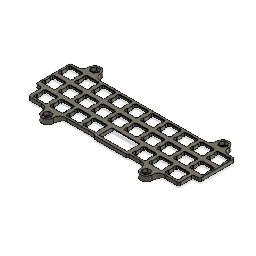
Alpha28PlateCase5mm v2 (Autodesk Fusion 360 design; units mm, degrees)
Autodesk Fusion 360 part; units mm, degrees
(part 1 of 6)
sketch "507b0d95479bd4c2c9a2277e45e886c67266d565_switch" plane through (0, 0, 0) normal (0, 1, 0) x (1, 0, 0)
  line L0 (189.063, 0.3128) -> (188.908, 0.2811)
  line L1 (190.215, 56.5838) -> (190.302, 56.4526)
  line L2 (190.444, 56.1728) -> (190.499, 56.0268)
  line L3 (189.063, 57.3525) -> (189.214, 57.3098)
  line L4 (1.3298, 0.4093) -> (1.1879, 0.474)
  line L5 (1.1879, 0.474) -> (1.0501, 0.5512)
  line L6 (1.6288, 0.3128) -> (1.4759, 0.3542)
  line L7 (190.302, 56.4526) -> (190.379, 56.315)
  line L8 (189.504, 57.1899) -> (189.64, 57.113)
  line L9 (190.444, 1.491) -> (190.379, 1.3491)
  line L10 (1.0501, 0.5512) -> (0.9192, 0.638)
  line L11 (190.572, 1.9444) -> (190.54, 1.7901)
  line L12 (190.117, 0.9577) -> (190.011, 0.842)
  line L13 (0.7965, 0.7359) -> (0.6808, 0.842)
  line L14 (0.5746, 0.9577) -> (0.4768, 1.0818)
  line L15 (0.248, 1.491) -> (0.1929, 1.6385)
  line L16 (1.4759, 0.3542) -> (1.3298, 0.4093)
  line L17 (189.771, 57.0258) -> (189.895, 56.9281)
  line L18 (0.4768, 1.0818) -> (0.39, 1.2127)
  line L19 (0.9192, 0.638) -> (0.7965, 0.7359)
  line L20 (190.499, 1.6385) -> (190.444, 1.491)
  line L21 (189.771, 0.638) -> (189.64, 0.5512)
  line L22 (190.572, 55.7209) -> (190.59, 55.5639)
  line L23 (190.379, 56.315) -> (190.444, 56.1728)
  line L24 (0.1929, 1.6385) -> (0.1502, 1.7901)
  line L25 (189.214, 57.3098) -> (189.362, 57.2548)
  line L26 (188.908, 57.3828) -> (189.063, 57.3525)
  line L27 (189.895, 56.9281) -> (190.011, 56.8219)
  line L28 (189.64, 57.113) -> (189.771, 57.0258)
  line L29 (190.117, 56.7062) -> (190.215, 56.5838)
  line L30 (190.499, 56.0268) -> (190.54, 55.874)
  line L31 (189.895, 0.7359) -> (189.771, 0.638)
  line L32 (189.214, 0.3542) -> (189.063, 0.3128)
  line L33 (0.6808, 0.842) -> (0.5746, 0.9577)
  line L34 (188.597, 0.2563) -> (2.096, 0.2577)
  line L35 (189.362, 0.4093) -> (189.214, 0.3542)
  line L36 (190.011, 56.8219) -> (190.117, 56.7062)
  line L37 (189.504, 0.474) -> (189.362, 0.4093)
  line L38 (190.596, 2.2572) -> (190.59, 2.1001)
  line L39 (2.096, 0.2577) -> (1.9389, 0.2632)
  line L40 (188.753, 57.4008) -> (188.908, 57.3828)
  line L41 (190.59, 55.5639) -> (190.596, 55.4069)
  line L42 (190.59, 2.1001) -> (190.572, 1.9444)
  line L43 (190.596, 55.4069) -> (190.596, 2.2572)
  line L44 (2.096, 57.4075) -> (188.597, 57.4075)
  line L45 (91.3197, 16.2319) -> (91.3197, 15.3128)
  line L46 (0.1502, 55.874) -> (0.1929, 56.0268)
  line L47 (0.1199, 1.9444) -> (0.102, 2.1001)
  line L48 (97.8711, 2.7823) -> (111.87, 2.7823)
  line L49 (0.3128, 56.315) -> (0.39, 56.4526)
  line L50 (0.3128, 1.3491) -> (0.248, 1.491)
  line L51 (115.12, 2.0326) -> (118.42, 2.0326)
  line L52 (0.248, 56.1728) -> (0.3128, 56.315)
  line L53 (97.8711, 6.8819) -> (97.0703, 6.8819)
  line L54 (190.302, 1.2127) -> (190.215, 1.0818)
  line L55 (188.597, 57.4075) -> (188.753, 57.4008)
  line L56 (112.671, 3.7827) -> (112.671, 6.8819)
  line L57 (188.753, 0.2632) -> (188.597, 0.2563)
  line L58 (190.54, 55.874) -> (190.572, 55.7209)
  line L59 (111.87, 2.7823) -> (111.87, 3.7827)
  line L60 (111.87, 6.8819) -> (111.87, 7.4827)
  line L61 (97.0703, 6.8819) -> (97.0703, 3.7827)
  line L62 (97.8711, 16.7817) -> (97.8711, 15.7827)
  line L63 (113.396, 3.0138) -> (115.12, 3.0138)
  line L64 (190.379, 1.3491) -> (190.302, 1.2127)
  line L65 (0.6808, 56.8219) -> (0.7965, 56.9281)
  line L66 (96.3454, 12.0826) -> (96.3454, 15.3128)
  line L67 (0.0951, 55.4069) -> (0.102, 55.5639)
  line L68 (1.9389, 57.4008) -> (2.096, 57.4075)
  line L69 (0.39, 1.2127) -> (0.3128, 1.3491)
  line L70 (0.1502, 1.7901) -> (0.1199, 1.9444)
  line L71 (190.215, 1.0818) -> (190.117, 0.9577)
  line L72 (190.54, 1.7901) -> (190.499, 1.6385)
  line L73 (94.6203, 2.0326) -> (94.6203, 3.0138)
  line L74 (189.362, 57.2548) -> (189.504, 57.1899)
  line L75 (96.3454, 15.3128) -> (94.6203, 15.3128)
  line L76 (111.87, 7.4827) -> (113.396, 7.4827)
  line L77 (1.3298, 57.2548) -> (1.4759, 57.3098)
  line L78 (190.011, 0.842) -> (189.895, 0.7359)
  line L79 (96.3454, 7.4827) -> (97.8711, 7.4827)
  line L80 (0.102, 2.1001) -> (0.0951, 2.2572)
  line L81 (1.1879, 57.1899) -> (1.3298, 57.2548)
  line L82 (97.8711, 7.4827) -> (97.8711, 6.8819)
  line L83 (1.9389, 0.2632) -> (1.7818, 0.2811)
  line L84 (118.42, 2.0326) -> (118.42, 3.0138)
  line L85 (0.5746, 56.7062) -> (0.6808, 56.8219)
  line L86 (1.7818, 57.3828) -> (1.9389, 57.4008)
  line L87 (97.8711, 12.0826) -> (96.3454, 12.0826)
  line L88 (189.64, 0.5512) -> (189.504, 0.474)
  line L89 (0.0951, 2.2572) -> (0.0951, 55.4069)
  line L90 (89.596, 9.2825) -> (89.596, 3.0138)
  line L91 (97.0703, 12.6821) -> (97.8711, 12.6821)
  line L92 (0.39, 56.4526) -> (0.4768, 56.5838)
  line L93 (94.6203, 16.2319) -> (91.3197, 16.2319)
  line L94 (188.908, 0.2811) -> (188.753, 0.2632)
  line L95 (1.7818, 0.2811) -> (1.6288, 0.3128)
  line L96 (113.396, 7.4827) -> (113.396, 3.0138)
  line L97 (1.0501, 57.113) -> (1.1879, 57.1899)
  line L98 (115.12, 3.0138) -> (115.12, 2.0326)
  line L99 (0.7965, 56.9281) -> (0.9192, 57.0258)
  line L100 (0.1929, 56.0268) -> (0.248, 56.1728)
  line L101 (111.87, 3.7827) -> (112.671, 3.7827)
  line L102 (0.4768, 56.5838) -> (0.5746, 56.7062)
  line L103 (88.7705, 9.2825) -> (89.596, 9.2825)
  line L104 (91.3197, 2.0326) -> (94.6203, 2.0326)
  line L105 (94.6203, 3.0138) -> (96.3454, 3.0138)
  line L106 (159.495, 3.7827) -> (160.296, 3.7827)
  line L107 (97.8711, 15.7827) -> (97.0703, 15.7827)
  line L108 (94.6203, 15.3128) -> (94.6203, 16.2319)
  line L109 (113.396, 12.0826) -> (111.87, 12.0826)
  line L110 (91.3197, 15.3128) -> (89.596, 15.3128)
  line L111 (112.671, 6.8819) -> (111.87, 6.8819)
  line L112 (159.495, 16.7817) -> (145.496, 16.7817)
  line L113 (178.545, 3.7827) -> (179.346, 3.7827)
  line L114 (144.695, 3.7827) -> (145.496, 3.7827)
  line L115 (126.446, 16.7817) -> (126.446, 15.7827)
  line L116 (112.671, 15.7827) -> (111.87, 15.7827)
  line L117 (125.645, 12.6821) -> (126.446, 12.6821)
  line L118 (145.496, 2.7823) -> (159.495, 2.7823)
  line L119 (159.495, 15.7827) -> (159.495, 16.7817)
  line L120 (111.87, 12.0826) -> (111.87, 12.6821)
  line L121 (164.546, 6.8819) -> (163.745, 6.8819)
  line L122 (120.146, 9.2825) -> (120.971, 9.2825)
  line L123 (89.596, 3.0138) -> (91.3197, 3.0138)
  line L124 (111.87, 12.6821) -> (112.671, 12.6821)
  line L125 (144.695, 15.7827) -> (144.695, 12.6821)
  line L126 (145.496, 3.7827) -> (145.496, 2.7823)
  line L127 (0.9192, 57.0258) -> (1.0501, 57.113)
  line L128 (126.446, 12.6821) -> (126.446, 6.8819)
  line L129 (160.296, 12.6821) -> (160.296, 15.7827)
  line L130 (89.596, 12.0826) -> (88.7705, 12.0826)
  line L131 (120.146, 15.3128) -> (118.42, 15.3128)
  line L132 (160.296, 15.7827) -> (159.495, 15.7827)
  line L133 (0.1199, 55.7209) -> (0.1502, 55.874)
  line L134 (163.745, 3.7827) -> (164.546, 3.7827)
  line L135 (115.12, 16.2319) -> (115.12, 15.3128)
  line L136 (126.446, 15.7827) -> (125.645, 15.7827)
  line L137 (118.42, 16.2319) -> (115.12, 16.2319)
  line L138 (163.745, 12.6821) -> (164.546, 12.6821)
  line L139 (178.545, 2.7823) -> (178.545, 3.7827)
  line L140 (164.546, 12.6821) -> (164.546, 6.8819)
  line L141 (159.495, 2.7823) -> (159.495, 3.7827)
  line L142 (179.346, 12.6821) -> (179.346, 15.7827)
  line L143 (178.545, 16.7817) -> (164.546, 16.7817)
  line L144 (97.8711, 12.6821) -> (97.8711, 12.0826)
  line L145 (88.7705, 12.0826) -> (88.7705, 9.2825)
  line L146 (111.87, 15.7827) -> (111.87, 16.7817)
  line L147 (164.546, 16.7817) -> (164.546, 15.7827)
  line L148 (97.0703, 3.7827) -> (97.8711, 3.7827)
  line L149 (91.3197, 3.0138) -> (91.3197, 2.0326)
  line L150 (89.596, 15.3128) -> (89.596, 12.0826)
  line L151 (96.3454, 3.0138) -> (96.3454, 7.4827)
  line L152 (178.545, 12.6821) -> (179.346, 12.6821)
  line L153 (97.8711, 3.7827) -> (97.8711, 2.7823)
  line L154 (97.0703, 15.7827) -> (97.0703, 12.6821)
  line L155 (1.4759, 57.3098) -> (1.6288, 57.3525)
  line L156 (1.6288, 57.3525) -> (1.7818, 57.3828)
  line L157 (145.496, 12.6821) -> (145.496, 6.8819)
  line L158 (160.296, 3.7827) -> (160.296, 6.8819)
  line L159 (145.496, 6.8819) -> (144.695, 6.8819)
  line L160 (159.495, 6.8819) -> (159.495, 12.6821)
  line L161 (159.495, 12.6821) -> (160.296, 12.6821)
  line L162 (120.146, 3.0138) -> (120.146, 9.2825)
  line L163 (164.546, 3.7827) -> (164.546, 2.7823)
  line L164 (164.546, 2.7823) -> (178.545, 2.7823)
  line L165 (179.346, 3.7827) -> (179.346, 6.8819)
  line L166 (0.102, 55.5639) -> (0.1199, 55.7209)
  line L167 (140.445, 15.7827) -> (140.445, 16.7817)
  line L168 (69.2961, 16.7817) -> (69.2961, 15.7827)
  line L169 (49.4453, 12.6821) -> (50.2461, 12.6821)
  line L170 (126.446, 2.7823) -> (140.445, 2.7823)
  line L171 (50.2461, 3.7827) -> (50.2461, 2.7823)
  line L172 (179.346, 6.8819) -> (178.545, 6.8819)
  line L173 (125.645, 15.7827) -> (125.645, 12.6821)
  line L174 (125.645, 6.8819) -> (125.645, 3.7827)
  line L175 (83.2954, 12.6821) -> (84.0962, 12.6821)
  line L176 (163.745, 15.7827) -> (163.745, 12.6821)
  line L177 (64.2454, 2.7823) -> (64.2454, 3.7827)
  line L178 (125.645, 3.7827) -> (126.446, 3.7827)
  line L179 (112.671, 12.6821) -> (112.671, 15.7827)
  line L180 (64.2454, 16.7817) -> (50.2461, 16.7817)
  line L181 (64.2454, 3.7827) -> (65.0462, 3.7827)
  line L182 (30.3954, 3.7827) -> (31.196, 3.7827)
  line L183 (140.445, 16.7817) -> (126.446, 16.7817)
  line L184 (118.42, 15.3128) -> (118.42, 16.2319)
  line L185 (120.971, 9.2825) -> (120.971, 12.0826)
  line L186 (164.546, 15.7827) -> (163.745, 15.7827)
  line L187 (145.496, 15.7827) -> (144.695, 15.7827)
  line L188 (120.146, 12.0826) -> (120.146, 15.3128)
  line L189 (30.3954, 15.7827) -> (30.3954, 12.6821)
  line L190 (178.545, 6.8819) -> (178.545, 12.6821)
  line L191 (126.446, 6.8819) -> (125.645, 6.8819)
  line L192 (113.396, 15.3128) -> (113.396, 12.0826)
  line L193 (68.4953, 6.8819) -> (68.4953, 3.7827)
  line L194 (144.695, 6.8819) -> (144.695, 3.7827)
  line L195 (50.2461, 16.7817) -> (50.2461, 15.7827)
  line L196 (65.0462, 12.6821) -> (65.0462, 15.7827)
  line L197 (31.196, 12.6821) -> (31.196, 6.8819)
  line L198 (31.196, 15.7827) -> (30.3954, 15.7827)
  line L199 (68.4953, 3.7827) -> (69.2961, 3.7827)
  line L200 (141.246, 12.6821) -> (141.246, 15.7827)
  line L201 (144.695, 12.6821) -> (145.496, 12.6821)
  line L202 (141.246, 6.8819) -> (140.445, 6.8819)
  line L203 (50.2461, 15.7827) -> (49.4453, 15.7827)
  line L204 (31.196, 16.7817) -> (31.196, 15.7827)
  line L205 (31.196, 3.7827) -> (31.196, 2.7823)
  line L206 (140.445, 6.8819) -> (140.445, 12.6821)
  line L207 (111.87, 16.7817) -> (97.8711, 16.7817)
  line L208 (145.496, 16.7817) -> (145.496, 15.7827)
  line L209 (30.3954, 12.6821) -> (31.196, 12.6821)
  line L210 (69.2961, 15.7827) -> (68.4953, 15.7827)
  line L211 (68.4953, 15.7827) -> (68.4953, 12.6821)
  line L212 (49.4453, 3.7827) -> (50.2461, 3.7827)
  line L213 (140.445, 12.6821) -> (141.246, 12.6821)
  line L214 (178.545, 15.7827) -> (178.545, 16.7817)
  line L215 (160.296, 6.8819) -> (159.495, 6.8819)
  line L216 (141.246, 15.7827) -> (140.445, 15.7827)
  line L217 (179.346, 15.7827) -> (178.545, 15.7827)
  line L218 (115.12, 15.3128) -> (113.396, 15.3128)
  line L219 (83.2954, 3.7827) -> (84.0962, 3.7827)
  line L220 (84.0962, 3.7827) -> (84.0962, 6.8819)
  line L221 (118.42, 3.0138) -> (120.146, 3.0138)
  line L222 (120.971, 12.0826) -> (120.146, 12.0826)
  line L223 (31.196, 6.8819) -> (30.3954, 6.8819)
  line L224 (140.445, 3.7827) -> (141.246, 3.7827)
  line L225 (30.3954, 6.8819) -> (30.3954, 3.7827)
  line L226 (163.745, 6.8819) -> (163.745, 3.7827)
  line L227 (69.2961, 12.6821) -> (69.2961, 6.8819)
  line L228 (83.2954, 15.7827) -> (83.2954, 16.7817)
  line L229 (26.1455, 12.6821) -> (26.9462, 12.6821)
  line L230 (84.0962, 6.8819) -> (83.2954, 6.8819)
  line L231 (45.1954, 3.7827) -> (45.9962, 3.7827)
  line L232 (64.2454, 6.8819) -> (64.2454, 12.6821)
  line L233 (141.246, 3.7827) -> (141.246, 6.8819)
  line L234 (50.2461, 6.8819) -> (49.4453, 6.8819)
  line L235 (84.0962, 15.7827) -> (83.2954, 15.7827)
  line L236 (26.9462, 6.8819) -> (26.1455, 6.8819)
  line L237 (174.071, 21.8323) -> (188.07, 21.8323)
  line L238 (65.0462, 3.7827) -> (65.0462, 6.8819)
  line L239 (12.146, 3.7827) -> (12.146, 2.7823)
  line L240 (69.2961, 3.7827) -> (69.2961, 2.7823)
  line L241 (65.0462, 6.8819) -> (64.2454, 6.8819)
  line L242 (50.2461, 12.6821) -> (50.2461, 6.8819)
  line L243 (64.2454, 12.6821) -> (65.0462, 12.6821)
  line L244 (68.4953, 12.6821) -> (69.2961, 12.6821)
  line L245 (65.0462, 15.7827) -> (64.2454, 15.7827)
  line L246 (83.2954, 2.7823) -> (83.2954, 3.7827)
  line L247 (126.446, 3.7827) -> (126.446, 2.7823)
  line L248 (83.2954, 6.8819) -> (83.2954, 12.6821)
  line L249 (69.2961, 6.8819) -> (68.4953, 6.8819)
  line L250 (50.2461, 2.7823) -> (64.2454, 2.7823)
  line L251 (140.445, 2.7823) -> (140.445, 3.7827)
  line L252 (83.2954, 16.7817) -> (69.2961, 16.7817)
  line L253 (49.4453, 15.7827) -> (49.4453, 12.6821)
  line L254 (169.821, 22.8327) -> (169.821, 25.9319)
  line L255 (45.9962, 12.6821) -> (45.9962, 15.7827)
  line L256 (49.4453, 6.8819) -> (49.4453, 3.7827)
  line L257 (84.0962, 12.6821) -> (84.0962, 15.7827)
  line L258 (26.1455, 6.8819) -> (26.1455, 12.6821)
  line L259 (26.1455, 16.7817) -> (12.146, 16.7817)
  line L260 (26.9462, 12.6821) -> (26.9462, 15.7827)
  line L261 (45.9962, 3.7827) -> (45.9962, 6.8819)
  line L262 (69.2961, 2.7823) -> (83.2954, 2.7823)
  line L263 (64.2454, 15.7827) -> (64.2454, 16.7817)
  line L264 (12.146, 6.8819) -> (11.3454, 6.8819)
  line L265 (11.3454, 6.8819) -> (11.3454, 3.7827)
  line L266 (135.971, 35.8316) -> (135.971, 34.8327)
  line L267 (116.92, 34.8327) -> (116.119, 34.8327)
  line L268 (188.07, 21.8323) -> (188.07, 22.8327)
  line L269 (11.3454, 15.7827) -> (11.3454, 12.6821)
  line L270 (26.1455, 15.7827) -> (26.1455, 16.7817)
  line L271 (188.871, 25.9319) -> (188.07, 25.9319)
  line L272 (174.071, 31.7321) -> (174.071, 25.9319)
  line L273 (188.871, 34.8327) -> (188.07, 34.8327)
  line L274 (155.021, 35.8316) -> (155.021, 34.8327)
  line L275 (45.1954, 6.8819) -> (45.1954, 12.6821)
  line L276 (26.9462, 3.7827) -> (26.9462, 6.8819)
  line L277 (174.071, 35.8316) -> (174.071, 34.8327)
  line L278 (12.146, 2.7823) -> (26.1455, 2.7823)
  line L279 (154.22, 34.8327) -> (154.22, 31.7321)
  line L280 (31.196, 2.7823) -> (45.1954, 2.7823)
  line L281 (173.27, 25.9319) -> (173.27, 22.8327)
  line L282 (188.07, 31.7321) -> (188.871, 31.7321)
  line L283 (188.07, 22.8327) -> (188.871, 22.8327)
  line L284 (155.021, 34.8327) -> (154.22, 34.8327)
  line L285 (155.021, 25.9319) -> (154.22, 25.9319)
  line L286 (188.871, 31.7321) -> (188.871, 34.8327)
  line L287 (154.22, 31.7321) -> (155.021, 31.7321)
  line L288 (45.1954, 2.7823) -> (45.1954, 3.7827)
  line L289 (45.9962, 15.7827) -> (45.1954, 15.7827)
  line L290 (45.1954, 12.6821) -> (45.9962, 12.6821)
  line L291 (174.071, 22.8327) -> (174.071, 21.8323)
  line L292 (154.22, 22.8327) -> (155.021, 22.8327)
  line L293 (26.1455, 3.7827) -> (26.9462, 3.7827)
  line L294 (45.1954, 15.7827) -> (45.1954, 16.7817)
  line L295 (188.871, 22.8327) -> (188.871, 25.9319)
  line L296 (173.27, 22.8327) -> (174.071, 22.8327)
  line L297 (45.1954, 16.7817) -> (31.196, 16.7817)
  line L298 (154.22, 25.9319) -> (154.22, 22.8327)
  line L299 (26.9462, 15.7827) -> (26.1455, 15.7827)
  line L300 (155.021, 31.7321) -> (155.021, 25.9319)
  line L301 (155.021, 22.8327) -> (155.021, 21.8323)
  line L302 (174.071, 34.8327) -> (173.27, 34.8327)
  line L303 (155.021, 21.8323) -> (169.02, 21.8323)
  line L304 (45.9962, 6.8819) -> (45.1954, 6.8819)
  line L305 (188.07, 35.8316) -> (174.071, 35.8316)
  line L306 (188.07, 34.8327) -> (188.07, 35.8316)
  line L307 (173.27, 34.8327) -> (173.27, 31.7321)
  line L308 (11.3454, 3.7827) -> (12.146, 3.7827)
  line L309 (12.146, 15.7827) -> (11.3454, 15.7827)
  line L310 (169.02, 21.8323) -> (169.02, 22.8327)
  line L311 (26.1455, 2.7823) -> (26.1455, 3.7827)
  line L312 (12.146, 16.7817) -> (12.146, 15.7827)
  line L313 (188.07, 25.9319) -> (188.07, 31.7321)
  line L314 (12.146, 12.6821) -> (12.146, 6.8819)
  line L315 (173.27, 31.7321) -> (174.071, 31.7321)
  line L316 (169.02, 22.8327) -> (169.821, 22.8327)
  line L317 (11.3454, 12.6821) -> (12.146, 12.6821)
  line L318 (174.071, 25.9319) -> (173.27, 25.9319)
  line L319 (169.02, 35.8316) -> (155.021, 35.8316)
  line L320 (112.67, 25.9319) -> (111.869, 25.9319)
  line L321 (149.97, 35.8316) -> (135.971, 35.8316)
  line L322 (149.97, 31.7321) -> (150.771, 31.7321)
  line L323 (135.17, 25.9319) -> (135.17, 22.8327)
  line L324 (78.8211, 25.9319) -> (78.0203, 25.9319)
  line L325 (135.971, 25.9319) -> (135.17, 25.9319)
  line L326 (97.8697, 25.9319) -> (97.0703, 25.9319)
  line L327 (169.02, 34.8327) -> (169.02, 35.8316)
  line L328 (97.0703, 22.8327) -> (97.8697, 22.8327)
  line L329 (112.67, 31.7321) -> (112.67, 34.8327)
  line L330 (130.92, 31.7321) -> (131.721, 31.7321)
  line L331 (130.92, 21.8323) -> (130.92, 22.8327)
  line L332 (135.17, 22.8327) -> (135.971, 22.8327)
  line L333 (116.92, 22.8327) -> (116.92, 21.8323)
  line L334 (111.869, 22.8327) -> (112.67, 22.8327)
  line L335 (116.92, 31.7321) -> (116.92, 25.9319)
  line L336 (97.8697, 34.8327) -> (97.0703, 34.8327)
  line L337 (116.119, 22.8327) -> (116.92, 22.8327)
  line L338 (150.771, 22.8327) -> (150.771, 25.9319)
  line L339 (130.92, 22.8327) -> (131.721, 22.8327)
  line L340 (169.821, 31.7321) -> (169.821, 34.8327)
  line L341 (131.721, 31.7321) -> (131.721, 34.8327)
  line L342 (169.02, 31.7321) -> (169.821, 31.7321)
  line L343 (97.8697, 21.8323) -> (111.869, 21.8323)
  line L344 (97.8697, 35.8316) -> (97.8697, 34.8327)
  line L345 (150.771, 31.7321) -> (150.771, 34.8327)
  line L346 (111.869, 25.9319) -> (111.869, 31.7321)
  line L347 (131.721, 22.8327) -> (131.721, 25.9319)
  line L348 (149.97, 34.8327) -> (149.97, 35.8316)
  line L349 (116.92, 35.8316) -> (116.92, 34.8327)
  line L350 (150.771, 25.9319) -> (149.97, 25.9319)
  line L351 (111.869, 21.8323) -> (111.869, 22.8327)
  line L352 (135.971, 21.8323) -> (149.97, 21.8323)
  line L353 (135.17, 31.7321) -> (135.971, 31.7321)
  line L354 (149.97, 21.8323) -> (149.97, 22.8327)
  line L355 (97.0703, 25.9319) -> (97.0703, 22.8327)
  line L356 (97.0703, 34.8327) -> (97.0703, 31.7321)
  line L357 (150.771, 34.8327) -> (149.97, 34.8327)
  line L358 (149.97, 22.8327) -> (150.771, 22.8327)
  line L359 (149.97, 25.9319) -> (149.97, 31.7321)
  line L360 (116.92, 21.8323) -> (130.92, 21.8323)
  line L361 (97.8697, 22.8327) -> (97.8697, 21.8323)
  line L362 (111.869, 31.7321) -> (112.67, 31.7321)
  line L363 (97.0703, 31.7321) -> (97.8697, 31.7321)
  line L364 (130.92, 25.9319) -> (130.92, 31.7321)
  line L365 (116.119, 25.9319) -> (116.119, 22.8327)
  line L366 (130.92, 35.8316) -> (116.92, 35.8316)
  line L367 (135.971, 31.7321) -> (135.971, 25.9319)
  line L368 (116.119, 34.8327) -> (116.119, 31.7321)
  line L369 (131.721, 34.8327) -> (130.92, 34.8327)
  line L370 (135.971, 22.8327) -> (135.971, 21.8323)
  line L371 (135.17, 34.8327) -> (135.17, 31.7321)
  line L372 (130.92, 34.8327) -> (130.92, 35.8316)
  line L373 (116.119, 31.7321) -> (116.92, 31.7321)
  line L374 (135.971, 34.8327) -> (135.17, 34.8327)
  line L375 (169.821, 25.9319) -> (169.02, 25.9319)
  line L376 (112.67, 22.8327) -> (112.67, 25.9319)
  line L377 (131.721, 25.9319) -> (130.92, 25.9319)
  line L378 (97.8697, 31.7321) -> (97.8697, 25.9319)
  line L379 (54.7204, 35.8316) -> (40.7211, 35.8316)
  line L380 (169.821, 34.8327) -> (169.02, 34.8327)
  line L381 (54.7204, 21.8323) -> (54.7204, 22.8327)
  line L382 (169.02, 25.9319) -> (169.02, 31.7321)
  line L383 (116.92, 25.9319) -> (116.119, 25.9319)
  line L384 (93.6198, 22.8327) -> (93.6198, 25.9319)
  line L385 (40.7211, 31.7321) -> (40.7211, 25.9319)
  line L386 (78.0203, 25.9319) -> (78.0203, 22.8327)
  line L387 (59.7711, 25.9319) -> (58.9703, 25.9319)
  line L388 (39.9203, 31.7321) -> (40.7211, 31.7321)
  line L389 (40.7211, 25.9319) -> (39.9203, 25.9319)
  line L390 (73.7704, 34.8327) -> (73.7704, 35.8316)
  line L391 (93.6198, 25.9319) -> (92.8204, 25.9319)
  line L392 (78.8211, 31.7321) -> (78.8211, 25.9319)
  line L393 (39.9203, 34.8327) -> (39.9203, 31.7321)
  line L394 (40.7211, 22.8327) -> (40.7211, 21.8323)
  line L395 (55.5212, 22.8327) -> (55.5212, 25.9319)
  line L396 (74.5712, 22.8327) -> (74.5712, 25.9319)
  line L397 (40.7211, 35.8316) -> (40.7211, 34.8327)
  line L398 (40.7211, 34.8327) -> (39.9203, 34.8327)
  line L399 (188.871, 41.8828) -> (188.871, 44.982)
  line L400 (73.7704, 31.7321) -> (74.5712, 31.7321)
  line L401 (112.67, 34.8327) -> (111.869, 34.8327)
  line L402 (74.5712, 34.8327) -> (73.7704, 34.8327)
  line L403 (39.9203, 22.8327) -> (40.7211, 22.8327)
  line L404 (40.7211, 21.8323) -> (54.7204, 21.8323)
  line L405 (55.5212, 34.8327) -> (54.7204, 34.8327)
  line L406 (73.7704, 21.8323) -> (73.7704, 22.8327)
  line L407 (93.6198, 34.8327) -> (92.8204, 34.8327)
  line L408 (92.8204, 25.9319) -> (92.8204, 31.7321)
  line L409 (59.7711, 31.7321) -> (59.7711, 25.9319)
  line L410 (73.7704, 35.8316) -> (59.7711, 35.8316)
  line L411 (59.7711, 22.8327) -> (59.7711, 21.8323)
  line L412 (58.9703, 31.7321) -> (59.7711, 31.7321)
  line L413 (111.869, 35.8316) -> (97.8697, 35.8316)
  line L414 (58.9703, 25.9319) -> (58.9703, 22.8327)
  line L415 (78.8211, 21.8323) -> (92.8204, 21.8323)
  line L416 (54.7204, 22.8327) -> (55.5212, 22.8327)
  line L417 (78.8211, 22.8327) -> (78.8211, 21.8323)
  line L418 (92.8204, 21.8323) -> (92.8204, 22.8327)
  line L419 (92.8204, 31.7321) -> (93.6198, 31.7321)
  line L420 (55.5212, 25.9319) -> (54.7204, 25.9319)
  line L421 (54.7204, 25.9319) -> (54.7204, 31.7321)
  line L422 (55.5212, 31.7321) -> (55.5212, 34.8327)
  line L423 (54.7204, 34.8327) -> (54.7204, 35.8316)
  line L424 (78.0203, 22.8327) -> (78.8211, 22.8327)
  line L425 (58.9703, 34.8327) -> (58.9703, 31.7321)
  line L426 (92.8204, 35.8316) -> (78.8211, 35.8316)
  line L427 (92.8204, 34.8327) -> (92.8204, 35.8316)
  line L428 (59.7711, 34.8327) -> (58.9703, 34.8327)
  line L429 (58.9703, 22.8327) -> (59.7711, 22.8327)
  line L430 (74.5712, 31.7321) -> (74.5712, 34.8327)
  line L431 (111.869, 34.8327) -> (111.869, 35.8316)
  line L432 (54.7204, 31.7321) -> (55.5212, 31.7321)
  line L433 (93.6198, 31.7321) -> (93.6198, 34.8327)
  line L434 (78.0203, 31.7321) -> (78.8211, 31.7321)
  line L435 (74.5712, 25.9319) -> (73.7704, 25.9319)
  line L436 (39.9203, 25.9319) -> (39.9203, 22.8327)
  line L437 (73.7704, 22.8327) -> (74.5712, 22.8327)
  line L438 (21.671, 35.8316) -> (21.671, 34.8327)
  line L439 (59.7711, 21.8323) -> (73.7704, 21.8323)
  line L440 (92.8204, 22.8327) -> (93.6198, 22.8327)
  line L441 (73.7704, 25.9319) -> (73.7704, 31.7321)
  line L442 (78.0203, 34.8327) -> (78.0203, 31.7321)
  line L443 (174.071, 41.8828) -> (174.071, 40.8824)
  line L444 (1.8204, 25.9319) -> (1.8204, 22.8327)
  line L445 (78.8211, 34.8327) -> (78.0203, 34.8327)
  line L446 (78.8211, 35.8316) -> (78.8211, 34.8327)
  line L447 (59.7711, 35.8316) -> (59.7711, 34.8327)
  line L448 (35.6704, 22.8327) -> (36.4712, 22.8327)
  line L449 (188.07, 54.8816) -> (174.071, 54.8816)
  line L450 (2.621, 34.8327) -> (1.8204, 34.8327)
  line L451 (16.6205, 25.9319) -> (16.6205, 31.7321)
  line L452 (21.671, 25.9319) -> (20.8704, 25.9319)
  line L453 (36.4712, 31.7321) -> (36.4712, 34.8327)
  line L454 (97.0703, 44.982) -> (97.0703, 41.8828)
  line L455 (174.071, 53.8826) -> (173.27, 53.8826)
  line L456 (155.021, 53.8826) -> (154.22, 53.8826)
  line L457 (173.27, 41.8828) -> (174.071, 41.8828)
  line L458 (1.8204, 31.7321) -> (2.621, 31.7321)
  line L459 (21.671, 31.7321) -> (21.671, 25.9319)
  line L460 (36.4712, 22.8327) -> (36.4712, 25.9319)
  line L461 (173.27, 53.8826) -> (173.27, 50.782)
  line L462 (35.6704, 21.8323) -> (35.6704, 22.8327)
  line L463 (2.621, 31.7321) -> (2.621, 25.9319)
  line L464 (16.6205, 35.8316) -> (2.621, 35.8316)
  line L465 (2.621, 35.8316) -> (2.621, 34.8327)
  line L466 (20.8704, 25.9319) -> (20.8704, 22.8327)
  line L467 (21.671, 34.8327) -> (20.8704, 34.8327)
  line L468 (2.621, 21.8323) -> (16.6205, 21.8323)
  line L469 (174.071, 44.982) -> (173.27, 44.982)
  line L470 (20.8704, 34.8327) -> (20.8704, 31.7321)
  line L471 (188.07, 50.782) -> (188.871, 50.782)
  line L472 (17.4212, 22.8327) -> (17.4212, 25.9319)
  line L473 (20.8704, 22.8327) -> (21.671, 22.8327)
  line L474 (188.871, 50.782) -> (188.871, 53.8826)
  line L475 (173.27, 44.982) -> (173.27, 41.8828)
  line L476 (35.6704, 25.9319) -> (35.6704, 31.7321)
  line L477 (155.021, 54.8816) -> (155.021, 53.8826)
  line L478 (20.8704, 31.7321) -> (21.671, 31.7321)
  line L479 (174.071, 40.8824) -> (188.07, 40.8824)
  line L480 (17.4212, 31.7321) -> (17.4212, 34.8327)
  line L481 (21.671, 22.8327) -> (21.671, 21.8323)
  line L482 (16.6205, 34.8327) -> (16.6205, 35.8316)
  line L483 (188.871, 44.982) -> (188.07, 44.982)
  line L484 (188.07, 40.8824) -> (188.07, 41.8828)
  line L485 (35.6704, 35.8316) -> (21.671, 35.8316)
  line L486 (174.071, 50.782) -> (174.071, 44.982)
  line L487 (188.871, 53.8826) -> (188.07, 53.8826)
  line L488 (155.021, 50.782) -> (155.021, 44.982)
  line L489 (188.07, 44.982) -> (188.07, 50.782)
  line L490 (21.671, 21.8323) -> (35.6704, 21.8323)
  line L491 (17.4212, 34.8327) -> (16.6205, 34.8327)
  line L492 (16.6205, 31.7321) -> (17.4212, 31.7321)
  line L493 (36.4712, 25.9319) -> (35.6704, 25.9319)
  line L494 (188.07, 53.8826) -> (188.07, 54.8816)
  line L495 (154.22, 50.782) -> (155.021, 50.782)
  line L496 (17.4212, 25.9319) -> (16.6205, 25.9319)
  line L497 (1.8204, 34.8327) -> (1.8204, 31.7321)
  line L498 (154.22, 53.8826) -> (154.22, 50.782)
  line L499 (2.621, 25.9319) -> (1.8204, 25.9319)
  line L500 (35.6704, 34.8327) -> (35.6704, 35.8316)
  line L501 (16.6205, 21.8323) -> (16.6205, 22.8327)
  line L502 (35.6704, 31.7321) -> (36.4712, 31.7321)
  line L503 (173.27, 50.782) -> (174.071, 50.782)
  line L504 (16.6205, 22.8327) -> (17.4212, 22.8327)
  line L505 (2.621, 22.8327) -> (2.621, 21.8323)
  line L506 (174.071, 54.8816) -> (174.071, 53.8826)
  line L507 (97.0703, 50.782) -> (97.8697, 50.782)
  line L508 (97.8697, 44.982) -> (97.0703, 44.982)
  line L509 (188.07, 41.8828) -> (188.871, 41.8828)
  line L510 (36.4712, 34.8327) -> (35.6704, 34.8327)
  line L511 (1.8204, 22.8327) -> (2.621, 22.8327)
  line L512 (116.92, 50.782) -> (116.92, 44.982)
  line L513 (116.119, 44.982) -> (116.119, 41.8828)
  line L514 (150.771, 44.982) -> (149.97, 44.982)
  line L515 (130.92, 54.8816) -> (116.92, 54.8816)
  line L516 (116.92, 54.8816) -> (116.92, 53.8826)
  line L517 (149.97, 44.982) -> (149.97, 50.782)
  line L518 (97.0703, 41.8828) -> (97.8697, 41.8828)
  line L519 (169.02, 41.8828) -> (169.821, 41.8828)
  line L520 (169.821, 53.8826) -> (169.02, 53.8826)
  line L521 (169.02, 54.8816) -> (155.021, 54.8816)
  line L522 (150.771, 53.8826) -> (149.97, 53.8826)
  line L523 (149.97, 53.8826) -> (149.97, 54.8816)
  line L524 (169.821, 41.8828) -> (169.821, 44.982)
  line L525 (135.971, 40.8824) -> (149.97, 40.8824)
  line L526 (150.771, 41.8828) -> (150.771, 44.982)
  line L527 (155.021, 44.982) -> (154.22, 44.982)
  line L528 (130.92, 50.782) -> (131.721, 50.782)
  line L529 (131.721, 53.8826) -> (130.92, 53.8826)
  line L530 (97.8697, 54.8816) -> (97.8697, 53.8826)
  line L531 (154.22, 41.8828) -> (155.021, 41.8828)
  line L532 (149.97, 54.8816) -> (135.971, 54.8816)
  line L533 (116.119, 41.8828) -> (116.92, 41.8828)
  line L534 (149.97, 50.782) -> (150.771, 50.782)
  line L535 (135.971, 50.782) -> (135.971, 44.982)
  line L536 (131.721, 50.782) -> (131.721, 53.8826)
  line L537 (155.021, 40.8824) -> (169.02, 40.8824)
  line L538 (116.119, 50.782) -> (116.92, 50.782)
  line L539 (97.8697, 50.782) -> (97.8697, 44.982)
  line L540 (149.97, 40.8824) -> (149.97, 41.8828)
  line L541 (135.17, 50.782) -> (135.971, 50.782)
  line L542 (131.721, 44.982) -> (130.92, 44.982)
  line L543 (135.17, 44.982) -> (135.17, 41.8828)
  line L544 (130.92, 44.982) -> (130.92, 50.782)
  line L545 (97.8697, 53.8826) -> (97.0703, 53.8826)
  line L546 (130.92, 53.8826) -> (130.92, 54.8816)
  line L547 (135.971, 44.982) -> (135.17, 44.982)
  line L548 (169.02, 50.782) -> (169.821, 50.782)
  line L549 (169.02, 44.982) -> (169.02, 50.782)
  line L550 (116.92, 40.8824) -> (130.92, 40.8824)
  line L551 (130.92, 41.8828) -> (131.721, 41.8828)
  line L552 (97.8697, 41.8828) -> (97.8697, 40.8824)
  line L553 (135.971, 53.8826) -> (135.17, 53.8826)
  line L554 (155.021, 41.8828) -> (155.021, 40.8824)
  line L555 (116.92, 53.8826) -> (116.119, 53.8826)
  line L556 (116.92, 44.982) -> (116.119, 44.982)
  line L557 (131.721, 41.8828) -> (131.721, 44.982)
  line L558 (116.119, 53.8826) -> (116.119, 50.782)
  line L559 (149.97, 41.8828) -> (150.771, 41.8828)
  line L560 (135.971, 41.8828) -> (135.971, 40.8824)
  line L561 (97.0703, 53.8826) -> (97.0703, 50.782)
  line L562 (39.9203, 53.8826) -> (39.9203, 50.782)
  line L563 (135.17, 41.8828) -> (135.971, 41.8828)
  line L564 (154.22, 44.982) -> (154.22, 41.8828)
  line L565 (150.771, 50.782) -> (150.771, 53.8826)
  line L566 (116.92, 41.8828) -> (116.92, 40.8824)
  line L567 (169.02, 40.8824) -> (169.02, 41.8828)
  line L568 (130.92, 40.8824) -> (130.92, 41.8828)
  line L569 (169.821, 44.982) -> (169.02, 44.982)
  line L570 (40.7211, 41.8828) -> (40.7211, 40.8824)
  line L571 (73.7704, 40.8824) -> (73.7704, 41.8828)
  line L572 (135.971, 54.8816) -> (135.971, 53.8826)
  line L573 (135.17, 53.8826) -> (135.17, 50.782)
  line L574 (169.02, 53.8826) -> (169.02, 54.8816)
  line L575 (169.821, 50.782) -> (169.821, 53.8826)
  line L576 (54.7204, 50.782) -> (55.5212, 50.782)
  line L577 (59.7711, 41.8828) -> (59.7711, 40.8824)
  line L578 (112.67, 50.782) -> (112.67, 53.8826)
  line L579 (92.8204, 53.8826) -> (92.8204, 54.8816)
  line L580 (93.6198, 41.8828) -> (93.6198, 44.982)
  line L581 (111.869, 54.8816) -> (97.8697, 54.8816)
  line L582 (39.9203, 44.982) -> (39.9203, 41.8828)
  line L583 (78.8211, 53.8826) -> (78.0203, 53.8826)
  line L584 (78.0203, 41.8828) -> (78.8211, 41.8828)
  line L585 (92.8204, 40.8824) -> (92.8204, 41.8828)
  line L586 (78.0203, 44.982) -> (78.0203, 41.8828)
  line L587 (93.6198, 44.982) -> (92.8204, 44.982)
  line L588 (40.7211, 54.8816) -> (40.7211, 53.8826)
  line L589 (21.671, 41.8828) -> (21.671, 40.8824)
  line L590 (73.7704, 44.982) -> (73.7704, 50.782)
  line L591 (21.671, 40.8824) -> (35.6704, 40.8824)
  line L592 (58.9703, 50.782) -> (59.7711, 50.782)
  line L593 (78.0203, 53.8826) -> (78.0203, 50.782)
  line L594 (59.7711, 44.982) -> (58.9703, 44.982)
  line L595 (112.67, 53.8826) -> (111.869, 53.8826)
  line L596 (39.9203, 41.8828) -> (40.7211, 41.8828)
  line L597 (74.5712, 41.8828) -> (74.5712, 44.982)
  line L598 (111.869, 50.782) -> (112.67, 50.782)
  line L599 (54.7204, 41.8828) -> (55.5212, 41.8828)
  line L600 (55.5212, 41.8828) -> (55.5212, 44.982)
  line L601 (111.869, 44.982) -> (111.869, 50.782)
  line L602 (92.8204, 54.8816) -> (78.8211, 54.8816)
  line L603 (39.9203, 50.782) -> (40.7211, 50.782)
  line L604 (93.6198, 50.782) -> (93.6198, 53.8826)
  line L605 (59.7711, 40.8824) -> (73.7704, 40.8824)
  line L606 (78.8211, 40.8824) -> (92.8204, 40.8824)
  line L607 (73.7704, 50.782) -> (74.5712, 50.782)
  line L608 (78.8211, 54.8816) -> (78.8211, 53.8826)
  line L609 (92.8204, 44.982) -> (92.8204, 50.782)
  line L610 (78.8211, 50.782) -> (78.8211, 44.982)
  line L611 (59.7711, 54.8816) -> (59.7711, 53.8826)
  line L612 (59.7711, 50.782) -> (59.7711, 44.982)
  line L613 (73.7704, 53.8826) -> (73.7704, 54.8816)
  line L614 (92.8204, 50.782) -> (93.6198, 50.782)
  line L615 (58.9703, 44.982) -> (58.9703, 41.8828)
  line L616 (74.5712, 53.8826) -> (73.7704, 53.8826)
  line L617 (93.6198, 53.8826) -> (92.8204, 53.8826)
  line L618 (111.869, 40.8824) -> (111.869, 41.8828)
  line L619 (40.7211, 44.982) -> (39.9203, 44.982)
  line L620 (78.8211, 44.982) -> (78.0203, 44.982)
  line L621 (111.869, 53.8826) -> (111.869, 54.8816)
  line L622 (59.7711, 53.8826) -> (58.9703, 53.8826)
  line L623 (40.7211, 40.8824) -> (54.7204, 40.8824)
  line L624 (78.0203, 50.782) -> (78.8211, 50.782)
  line L625 (112.67, 41.8828) -> (112.67, 44.982)
  line L626 (54.7204, 40.8824) -> (54.7204, 41.8828)
  line L627 (97.8697, 40.8824) -> (111.869, 40.8824)
  line L628 (40.7211, 53.8826) -> (39.9203, 53.8826)
  line L629 (58.9703, 53.8826) -> (58.9703, 50.782)
  line L630 (111.869, 41.8828) -> (112.67, 41.8828)
  line L631 (74.5712, 50.782) -> (74.5712, 53.8826)
  line L632 (112.67, 44.982) -> (111.869, 44.982)
  line L633 (74.5712, 44.982) -> (73.7704, 44.982)
  line L634 (78.8211, 41.8828) -> (78.8211, 40.8824)
  line L635 (58.9703, 41.8828) -> (59.7711, 41.8828)
  line L636 (92.8204, 41.8828) -> (93.6198, 41.8828)
  line L637 (73.7704, 41.8828) -> (74.5712, 41.8828)
  line L638 (40.7211, 50.782) -> (40.7211, 44.982)
  line L639 (73.7704, 54.8816) -> (59.7711, 54.8816)
  line L640 (35.6704, 40.8824) -> (35.6704, 41.8828)
  line L641 (16.6205, 53.8826) -> (16.6205, 54.8816)
  line L642 (21.671, 44.982) -> (20.8704, 44.982)
  line L643 (2.621, 44.982) -> (1.8204, 44.982)
  line L644 (55.5212, 44.982) -> (54.7204, 44.982)
  line L645 (35.6704, 44.982) -> (35.6704, 50.782)
  line L646 (2.621, 50.782) -> (2.621, 44.982)
  line L647 (55.5212, 53.8826) -> (54.7204, 53.8826)
  line L648 (20.8704, 41.8828) -> (21.671, 41.8828)
  line L649 (17.4212, 41.8828) -> (17.4212, 44.982)
  line L650 (35.6704, 54.8816) -> (21.671, 54.8816)
  line L651 (54.7204, 53.8826) -> (54.7204, 54.8816)
  line L652 (16.6205, 50.782) -> (17.4212, 50.782)
  line L653 (54.7204, 54.8816) -> (40.7211, 54.8816)
  line L654 (1.8204, 53.8826) -> (1.8204, 50.782)
  line L655 (1.8204, 41.8828) -> (2.621, 41.8828)
  line L656 (17.4212, 50.782) -> (17.4212, 53.8826)
  line L657 (35.6704, 41.8828) -> (36.4712, 41.8828)
  line L658 (17.4212, 53.8826) -> (16.6205, 53.8826)
  line L659 (35.6704, 50.782) -> (36.4712, 50.782)
  line L660 (21.671, 50.782) -> (21.671, 44.982)
  line L661 (16.6205, 41.8828) -> (17.4212, 41.8828)
  line L662 (2.621, 53.8826) -> (1.8204, 53.8826)
  line L663 (2.621, 41.8828) -> (2.621, 40.8824)
  line L664 (2.621, 40.8824) -> (16.6205, 40.8824)
  line L665 (17.4212, 44.982) -> (16.6205, 44.982)
  line L666 (36.4712, 41.8828) -> (36.4712, 44.982)
  line L667 (54.7204, 44.982) -> (54.7204, 50.782)
  line L668 (36.4712, 44.982) -> (35.6704, 44.982)
  line L669 (21.671, 53.8826) -> (20.8704, 53.8826)
  line L670 (55.5212, 50.782) -> (55.5212, 53.8826)
  line L671 (16.6205, 40.8824) -> (16.6205, 41.8828)
  line L672 (1.8204, 44.982) -> (1.8204, 41.8828)
  line L673 (35.6704, 53.8826) -> (35.6704, 54.8816)
  line L674 (2.621, 54.8816) -> (2.621, 53.8826)
  line L675 (36.4712, 50.782) -> (36.4712, 53.8826)
  line L676 (16.6205, 44.982) -> (16.6205, 50.782)
  line L677 (16.6205, 54.8816) -> (2.621, 54.8816)
  line L678 (1.8204, 50.782) -> (2.621, 50.782)
  line L679 (20.8704, 53.8826) -> (20.8704, 50.782)
  line L680 (21.671, 54.8816) -> (21.671, 53.8826)
  line L681 (20.8704, 44.982) -> (20.8704, 41.8828)
  line L682 (20.8704, 50.782) -> (21.671, 50.782)
  line L683 (36.4712, 53.8826) -> (35.6704, 53.8826)
extrude "Extrude1" add sketch "507b0d95479bd4c2c9a2277e45e886c67266d565_switch" against normal blind 4
sketch "Sketch2" plane through (0, 0, 0) normal (0, 1, 0) x (-1, 0, 0)
  line L0 (-188.597, -57.4075) -> (-2.096, -57.4075)
  circle A0 centre (-169.5819, -64.9075) radius 2.6
  line L1 (-169.5819, -64.9075) -> (-169.5819, -57.4075) construction
  line L2 (-171.8315, -68.9414) -> (-167.2132, -68.8727)
  line L3 (-167.2132, -68.8727) -> (-164.9636, -64.8387)
  line L4 (-164.9636, -64.8387) -> (-167.3323, -60.8736)
  line L5 (-167.3323, -60.8736) -> (-171.9506, -60.9423)
  line L6 (-171.9506, -60.9423) -> (-174.2002, -64.9763)
  line L7 (-174.2002, -64.9763) -> (-171.8315, -68.9414)
  line L8 (-154.9924, -57.4075) -> (-162.7837, -57.4075)
  line L9 (-162.7837, -57.4075) -> (-162.7837, -64.9763)
  spline S0 degree 2 poles (-154.9924, -57.4075) (-162.7837, -57.4075) (-162.7837, -64.9763) knots 0 0 0 1 1 1
  line L10 (-169.5819, -64.9075) -> (-169.5819, -64)
  line L11 (-169.5819, -64) -> (-169.5819, -69) construction
  spline S1 degree 2 poles (-184.1714, -57.4075) (-176.3801, -57.4075) (-176.3801, -64.9763) knots 0 0 0 1 1 1
  line L12 (-184.1714, -57.4075) -> (-176.3801, -57.4075)
  line L13 (-176.3801, -57.4075) -> (-176.3801, -64.9763)
  arc A1 (-176.3801, -64.9763) -> (-162.7837, -64.9763) centre (-169.5819, -64.5335) ccw
  line L14 (-0.0951, -2.2572) -> (-0.0951, -55.4069)
  line L15 (-190.596, -55.4069) -> (-190.596, -2.2572)
  line L16 (-188.597, -0.2563) -> (-2.096, -0.2577)
  line L17 (-0.0951, -28.8321) -> (-190.596, -28.8321) construction
  line L18 (-95.3465, -57.4075) -> (-95.3465, -0.257) construction
  line L19 (-21.1111, -64) -> (-21.1111, -69) construction
  line L20 (-23.4798, -68.8727) -> (-25.7294, -64.8387)
  line L21 (-21.1111, -64.9075) -> (-21.1111, -57.4075) construction
  line L22 (-21.1111, -64.9075) -> (-21.1111, -64)
  line L23 (-23.3607, -60.8736) -> (-18.7424, -60.9423)
  line L24 (-18.7424, -60.9423) -> (-16.4928, -64.9763)
  spline S2 degree 2 poles (-6.5216, -57.4075) (-14.3129, -57.4075) (-14.3129, -64.9763) knots 0 0 0 1 1 1
  line L25 (-6.5216, -57.4075) -> (-14.3129, -57.4075)
  line L26 (-14.3129, -57.4075) -> (-14.3129, -64.9763)
  arc A2 (-27.9093, -64.9763) -> (-14.3129, -64.9763) centre (-21.1111, -64.5335) ccw
  spline S3 degree 2 poles (-35.7006, -57.4075) (-27.9093, -57.4075) (-27.9093, -64.9763) knots 0 0 0 1 1 1
  line L27 (-35.7006, -57.4075) -> (-27.9093, -57.4075)
  line L28 (-27.9093, -57.4075) -> (-27.9093, -64.9763)
  line L29 (-16.4928, -64.9763) -> (-18.8615, -68.9414)
  line L30 (-18.8615, -68.9414) -> (-23.4798, -68.8727)
  line L31 (-25.7294, -64.8387) -> (-23.3607, -60.8736)
  circle A3 centre (-21.1111, -64.9075) radius 2.6
  line L32 (-174.2002, -64.9763) -> (-176.3801, -64.9763) construction
  circle A4 centre (-152.5137, 7.2435) radius 2.6
  arc A5 (-145.716, 7.3123) -> (-159.3113, 7.3119) centre (-152.5137, 6.8699) ccw
  spline S4 degree 2 poles (-137.8078, -0.2567) (-145.7158, -0.2561) (-145.716, 7.3123) knots 0 0 0 1 1 1
  line L33 (-137.8078, -0.2567) -> (-145.7158, -0.2561)
  line L34 (-145.7158, -0.2561) -> (-145.716, 7.3123)
  line L35 (-147.8954, 7.3122) -> (-145.716, 7.3123) construction
  line L36 (-147.8954, 7.3122) -> (-150.2641, 11.2774)
  line L37 (-154.7632, 3.2095) -> (-150.145, 3.2783)
  line L38 (-150.145, 3.2783) -> (-147.8954, 7.3122)
  line L39 (-157.132, 7.1747) -> (-154.7632, 3.2095)
  line L40 (-152.5137, 7.2435) -> (-152.5136, 6.3362)
  line L41 (-150.2641, 11.2774) -> (-154.8824, 11.2086)
  line L42 (-154.8824, 11.2086) -> (-157.132, 7.1747)
  line L43 (-152.5136, 6.3362) -> (-152.5138, 11.3362) construction
  line L44 (-152.5137, 7.2435) -> (-152.5134, -0.2565) construction
  spline S5 degree 2 poles (-167.2191, -0.2575) (-159.3111, -0.2565) (-159.3113, 7.3119) knots 0 0 0 1 1 1
  line L45 (-167.2191, -0.2575) -> (-159.3111, -0.2565)
  line L46 (-159.3111, -0.2565) -> (-159.3113, 7.3119)
  line L47 (-42.7976, 7.3122) -> (-44.977, 7.3123) construction
  line L48 (-38.1794, 6.3362) -> (-38.1792, 11.3362) construction
  circle A6 centre (-38.1793, 7.2435) radius 2.6
  line L49 (-33.561, 7.1747) -> (-35.9298, 3.2095)
  line L50 (-40.4289, 11.2774) -> (-35.8106, 11.2086)
  line L51 (-35.8106, 11.2086) -> (-33.561, 7.1747)
  line L52 (-38.1793, 7.2435) -> (-38.1794, 6.3362)
  line L53 (-35.9298, 3.2095) -> (-40.548, 3.2783)
  line L54 (-40.548, 3.2783) -> (-42.7976, 7.3122)
  line L55 (-42.7976, 7.3122) -> (-40.4289, 11.2774)
  spline S6 degree 2 poles (-52.8852, -0.2567) (-44.9772, -0.2561) (-44.977, 7.3123) knots 0 0 0 1 1 1
  line L56 (-52.8852, -0.2567) -> (-44.9772, -0.2561)
  line L57 (-44.9772, -0.2561) -> (-44.977, 7.3123)
  line L58 (-38.1793, 7.2435) -> (-38.1796, -0.2565) construction
  arc A7 (-31.3817, 7.3119) -> (-44.977, 7.3123) centre (-38.1793, 6.8699) ccw
  spline S7 degree 2 poles (-23.4739, -0.2575) (-31.3819, -0.2565) (-31.3817, 7.3119) knots 0 0 0 1 1 1
  line L59 (-23.4739, -0.2575) -> (-31.3819, -0.2565)
  line L60 (-31.3819, -0.2565) -> (-31.3817, 7.3119)
  line L61 (-52.8852, -0.2567) -> (-53.3, -0.4)
  point P0 (-169.5819, -64.9075)
  point P1 (-162.7837, -57.4075)
  point P2 (-27.9093, -57.4075)
  point P3 (-21.1111, -64.9075)
  point P4 (-159.3111, -0.2565)
  point P5 (-152.5137, 7.2435)
  point P6 (-38.1793, 7.2435)
  point P7 (-31.3819, -0.2565)
  dimension "d5" = 5.2
  dimension "d52" = 7.5
  dimension "d54" = 4
  dimension "d66" = 5.2
  dimension "d67" = 7.5
  dimension "d68" = 4
  constraint coincident P0 A0.centre
  constraint coincident L0 L1.end
  constraint perpendicular L0 L1
  constraint coincident L0 L8.start
  constraint coincident P1 L8.end
  constraint parallel L1 L9
  constraint parallel L1 L10
  constraint parallel L10 L11
  constraint symmetric L1 L8.start S1.start
  constraint symmetric L1 L9.end S1.end
  constraint symmetric L1 S0 S1
  constraint midpoint L14 L17.start
  constraint midpoint L15 L17.end
  constraint midpoint L0 L18.start
  constraint midpoint L16 L18.end
  constraint symmetric P0 L18 P3
  constraint symmetric L1.end L18 L21.end
  constraint symmetric A0 L18 A3
  constraint symmetric L2.start L18 L29.end
  constraint symmetric L2.end L18 L20.start
  constraint symmetric L3.end L18 L20.end
  constraint symmetric L4.end L18 L23.start
  constraint symmetric L5.end L18 L23.end
  constraint symmetric L6.end L18 L24.end
  constraint symmetric P1 L18 P2
  constraint symmetric L8.start L18 S3.start
  constraint symmetric L9.end L18 A2.start
  constraint symmetric S0 L18 S3
  constraint symmetric L10.end L18 L19.start
  constraint symmetric L11.end L18 L19.end
  constraint symmetric S1.start L18 S2.start
  constraint symmetric S1.end L18 S2.end
  constraint symmetric S1 L18 S2
  constraint symmetric A1 L18 A2
  constraint perpendicular L13 L32
  constraint coincident P5 A4.centre
  constraint coincident P4 L45.end
  constraint parallel L44 L46
  constraint parallel L40 L44
  constraint parallel L40 L43
  constraint symmetric A5.end A5.start L44
  constraint symmetric S4 L44 S5
  constraint perpendicular L34 L35
  constraint coincident L16 S4.start
  constraint symmetric L18 P5 P6
  constraint symmetric L18 A5.end A7.start
  constraint symmetric L18 L40.end L48.start
  constraint symmetric L18 L43.end L48.end
  constraint symmetric L18 A5.start L47.end
  constraint symmetric L18 L35.start L47.start
  constraint symmetric L18 L37.end L53.end
  constraint symmetric L18 L37.start L49.end
  constraint symmetric L18 P4 P7
  constraint symmetric L18 L36.end L50.start
  constraint symmetric L18 L39.start L49.start
  constraint symmetric L18 L41.end L50.end
  constraint symmetric L18 L44.end L58.end
  constraint symmetric L18 A4 A6
  constraint symmetric L18 A5 A7
  constraint symmetric L18 S4 S6
  constraint symmetric L18 S5 S7
  constraint coincident L16 S7.start
  measures "d5" diameter of A0
  measures "d52" distance of P0 L1.end
  measures "d54" distance of P0 L7
  measures "d66" diameter of A4
  measures "d67" distance of P5 L44.end
  measures "d68" distance of P5 L36
extrude "Extrude2" add sketch "Sketch2" against normal blind 6 contours L0 S1 L12 L13 | L0 L9 L13 A1 | L0 L8 L9 S0 | L0 S3 L27 L28 | L0 L26 A2 L28 | L0 S2 L25 L26 | L2 L3 L4 L5 L6 L7 | L16 A5 L33 L34 L46 | L16 S5 L46 | S4 L33 L34 | L16 L56 L57 A7 L59 L60 L61 | S7 L59 L60 | S6 L56 L57 | L20 L23 L24 L29 L30 L31 | L36 L37 L38 L39 L41 L42 | L49 L50 L51 L53 L54 L55
chamfer "Chamfer2" distance 2 angle 45 4 edges at (21.1111, -6, -57.4075) (38.1805, -6, -0.2574) (152.4214, -6, -0.2566) (169.5819, -6, -57.4075)
extrude "Extrude3" cut sketch "Sketch2" against normal blind 4 contours L2 L3 L4 L5 L6 L7 | L20 L23 L24 L29 L30 L31 | L36 L37 L38 L39 L41 L42 | L49 L50 L51 L53 L54 L55